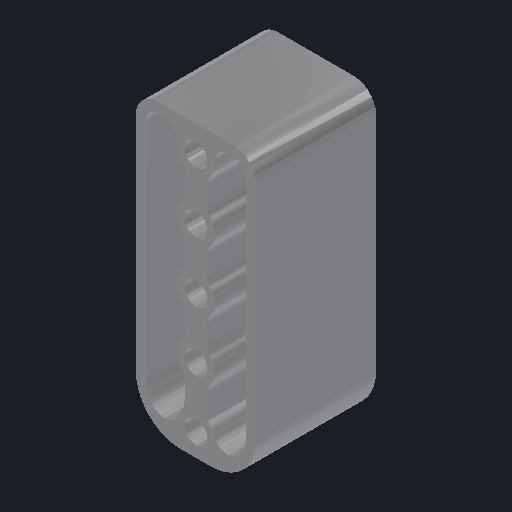
# Autodesk Inventor part: SDS LOWERING SPACER
Saved by Autodesk Inventor 2024.3 (Build 283343000, 343)
## iProperties
ILogicPurgeVersion: 0.0.0.0
OnSaveVersion: 3.5.0.0
OnSaveAssembly: COREAutomationManager
Category: _
Manager: _
Created: 2025-03-17
Part Number: SDS LOWERING SPACER
Checked By: 00
Engr Approved By: _
User Status: Work In Process
Material: Aluminum 7075
Description: STANDARD (mm)
Document SubType Name: Modeling
Mfg Approved By: John.Thibert
Designer: John.Thibert
Manufacturer: Standard
Standards Organization: Custom
Mass: 42.4696 g
Surface Area: 133.672 cm^2
Volume: 15.1137 cm^3
Density: 2.81 g/cm^3
Appearance: Aluminum - Polished
CN_MASS: 0.04
CN_SERVICEABLE: _
FIRST_DESCRIPTION: _
SECOND_DESCRIPTION: _
THIRD_DESCRIPTION: _
ModelCat: Uncategorized
MaterialName: Aluminum 7075
Subject: _
Author: John.Thibert
Keywords: -
Revision Number: A
Autodesk Inventor part; units mm, degrees
ref_plane "YZ Plane" through (0, 0, 0) normal (1, 0, 0) x (0, 1, 0)
ref_plane "XZ Plane" through (0, 0, 0) normal (0, 1, 0) x (-1, 0, 0)
ref_plane "XY Plane" through (0, 0, 0) normal (0, 0, 1) x (1, 0, 0)
sketch "Sketch2" plane through (0, 0, 0) normal (0, 0, 1) x (1, 0, 0)
  line L0 (-12.7, -30.6388) -> (12.7, -30.6388)
  line L1 (12.7, -30.6388) -> (12.7, 30.6388)
  line L2 (12.7, 30.6388) -> (-12.7, 30.6388)
  line L3 (-12.7, 30.6388) -> (-12.7, -30.6388)
  line L4 (-12.7, -30.6388) -> (12.7, 30.6388) construction
  line L5 (12.7, -30.6388) -> (-12.7, 30.6388) construction
  line L6 (0, 30.6388) -> (0, -30.6388) construction
  point P0 (0, 0)
  dimension "d0" = 25.4
  dimension "d1" = 61.2775
  constraints: 14 end point, 4 midpoint, 2 parallel, 1 horizontal, 1 perpendicular
  measures "d0" distance of L2.end L1.end
  measures "d1" distance of L1.end L0.end
extrude "Extrusion1" add sketch "Sketch2" along normal blind 25.4
sketch "Sketch3" plane through (0, 0, 25.4) normal (0, 0, 1) x (1, 0, 0)
  line L0 (-12.7, -30.6388) -> (12.7, -30.6388) construction
  point P0 (0, 0)
  point P1 (0, -25.8762)
  dimension "d5" = 4.7625
  constraints: 1 vertical alignment
  measures "d5" distance from line of L0 point (0, -25.876)
hole "Hole1" at (0, -25.8762, 25.4) direction (0, 0, -1) diameter 4.826 end through all start extended yes clearance for "Flat Head Machine Screw (82)" size "#10" standard "Ansi Unified Screw Threads"
fillet "Fillet1" radius 9.525 2 edges at (-12.7, -30.6388, 12.7) (12.7, -30.6388, 12.7)
pattern_linear "Rectangular Pattern1" count 5 spacing 12.7 along (0, 1, 0) of "Hole1"
sketch "Sketch4" plane through (0, 0, 25.4) normal (0, 0, 1) x (1, 0, 0)
  circle A0 centre (0, 24.9237) radius 2.413 projected
  circle A1 centre (0, 12.2237) radius 2.413 projected
  circle A2 centre (0, -0.4763) radius 2.413 projected
  circle A3 centre (0, -13.1762) radius 2.413 projected
  arc A4 (3.175, -30.6388) -> (12.7, -21.1137) centre (3.175, -21.1137) ccw projected
  line L0 (12.7, -21.1137) -> (12.7, 30.6388) projected
  line L1 (12.7, 30.6388) -> (-12.7, 30.6388) projected
  line L2 (-12.7, 30.6388) -> (-12.7, -21.1138) projected
  arc A5 (-12.7, -21.1138) -> (-3.175, -30.6388) centre (-3.175, -21.1138) ccw projected
  line L3 (-3.175, -30.6388) -> (3.175, -30.6388) projected
  circle A6 centre (0, -25.8762) radius 2.413 projected
  circle A7 centre (0, -25.8762) radius 3.9688
  circle A8 centre (0, -13.1762) radius 3.9688
  circle A9 centre (0, -0.4763) radius 3.9688
  circle A10 centre (0, 12.2237) radius 3.9688
  circle A11 centre (0, 24.9237) radius 3.9688
  line L4 (2.413, -22.7253) -> (2.413, -16.3272)
  line L5 (2.413, -10.0253) -> (2.413, -3.6272)
  line L6 (-2.413, -22.7253) -> (-2.413, -16.3272)
  line L7 (-2.413, -10.0253) -> (-2.413, -3.6272)
  line L8 (2.413, 2.6747) -> (2.413, 9.0728)
  line L9 (-2.413, 2.6747) -> (-2.413, 9.0728)
  line L10 (-2.413, 15.3747) -> (-2.413, 21.7728)
  line L11 (2.413, 15.3747) -> (2.413, 21.7728)
  arc A12 (-10.668, -21.1138) -> (-3.175, -28.6068) centre (-3.175, -21.1138) ccw
  line L12 (-10.668, -21.1138) -> (-10.668, 28.6068)
  line L13 (-10.668, 28.6068) -> (10.668, 28.6068)
  line L14 (10.668, 28.6068) -> (10.668, -21.1137)
  arc A13 (3.175, -28.6068) -> (10.668, -21.1137) centre (3.175, -21.1137) ccw
  line L15 (3.175, -28.6068) -> (-3.175, -28.6068)
  point P0 (0, 0)
  point P1 (1.4787, 28.6068)
  point P2 (2.8802, -28.6068)
  point P3 (-2.8802, -28.6068)
  point P4 (-1.4787, 28.6068)
  dimension "d16" = 7.9375
  dimension "d17" = 2.032
  constraints: 24 end point, 20 point on circle, 16 tangent, 7 centre point, 4 equal radius, 5 other
  measures "d16" diameter of A7
  measures "d17" distance between parallel lines of L2 L12
extrude "Extrusion2" cut sketch "Sketch4" against normal through all contours A7 L4 A8 L5 A9 L8 A10 L11 A11 L13 L14 A13 L15 | A7 L15 A12 L12 L13 A11 L10 A10 L9 A9 L7 A8 L6
fillet "Fillet2" radius 3.175 21 edges at (2.8802, -28.6068, 12.7) (-2.8802, -28.6068, 12.7) (-1.4787, 28.6068, 12.7) (1.4787, 28.6068, 12.7) (-10.668, 28.6068, 12.7) (10.668, 28.6068, 12.7) (2.413, -16.3272, 12.7) (2.413, -10.0253, 12.7) (2.413, -3.6272, 12.7) (2.413, 2.6747, 12.7) (2.413, 9.0728, 12.7) (2.413, 15.3747, 12.7) (2.413, 21.7728, 12.7) (-2.413, -16.3272, 12.7) (-2.413, -10.0253, 12.7) (-2.413, -3.6272, 12.7) (-2.413, 2.6747, 12.7) (-2.413, 9.0728, 12.7) (-2.413, 15.3747, 12.7) (-2.413, 21.7728, 12.7) (-2.413, -22.7253, 12.7)
fillet "Fillet3" radius 4.7625 2 edges at (12.7, 30.6388, 12.7) (-12.7, 30.6388, 12.7)
body "Solid1"
